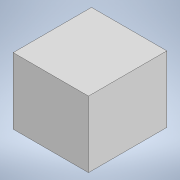
# Autodesk Inventor part: main_block
Saved by Autodesk Inventor 2021 (Build 250183000, 183)
## iProperties
Created: 2020-06-26
Part Number: main_block
Material: Generic
Document SubType Name: Modeling
Designer: Yatekii
Density: 1 g/cm^3
Appearance: Default
Author: Yatekii
Autodesk Inventor part; units mm, degrees
ref_plane "YZ Plane" through (0, 0, 0) normal (1, 0, 0) x (0, 1, 0)
ref_plane "XZ Plane" through (0, 0, 0) normal (0, 1, 0) x (-1, 0, 0)
ref_plane "XY Plane" through (0, 0, 0) normal (0, 0, 1) x (1, 0, 0)
sketch "Sketch2" plane through (0, 0, 0) normal (0, 1, 0) x (-1, 0, 0)
  line L0 (-12.5, -13) -> (12.5, -13)
  line L1 (12.5, -13) -> (12.5, 13)
  line L2 (12.5, 13) -> (-12.5, 13)
  line L3 (-12.5, 13) -> (-12.5, -13)
  line L4 (-12.5, -13) -> (12.5, 13) construction
  line L5 (12.5, -13) -> (-12.5, 13) construction
  point P0 (0, 0)
  dimension "d0" = 25
  dimension "d1" = 26
  constraints: 12 end point, 2 midpoint, 2 parallel, 1 horizontal, 1 perpendicular
  measures "d0" distance of L2.end L1.end
  measures "d1" distance of L1.end L0.end
extrude "Extrusion1" add sketch "Sketch2" along normal blind 22
body "Solid1"
